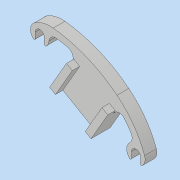
# Autodesk Inventor part: USBBreakoutHolder
Saved by Autodesk Inventor 2017 (Build 210142000, 142)
## iProperties
Created: 2019-07-16
Part Number: USBBreakoutHolder
Material: Generic
Document SubType Name: Modeling
Designer: techn
Density: 1 g/cm^3
Appearance: Default
Author: techn
Autodesk Inventor part; units mm, degrees
ref_plane "YZ Plane" through (0, 0, 0) normal (1, 0, 0) x (0, 1, 0)
ref_plane "XZ Plane" through (0, 0, 0) normal (0, 1, 0) x (-1, 0, 0)
ref_plane "XY Plane" through (0, 0, 0) normal (0, 0, 1) x (1, 0, 0)
sketch "Sketch1" plane through (0, 0, 0) normal (0, 0, 1) x (1, 0, 0)
  arc A0 (1.7145, 0) -> (-1.7145, 0) centre (0, 0) ccw
  arc A1 (38.0096, -20.955) -> (34.5806, -20.955) centre (36.2951, -20.955) ccw
  line L0 (0, 0) -> (36.5724, 0) construction
  line L1 (-1.7145, 0) -> (-1.7145, -3.0427)
  line L2 (1.7145, 0) -> (1.7145, -3.0427)
  line L3 (34.5806, -20.955) -> (34.5806, -23.9977)
  line L4 (38.0096, -20.955) -> (38.0096, -23.9977)
  line L5 (0, 0) -> (0, -41.91) construction
  arc A2 (29.1702, -5.2325) -> (5.0807, 4.6768) centre (0, -41.91) ccw
  arc A3 (5.0807, 4.6768) -> (-2.0016, 2.862) centre (3.9541, -5.6536) ccw
  arc A4 (39.5833, -19.7781) -> (29.1702, -5.2325) centre (8.8547, -30.7765) ccw
  arc A5 (4.8053, 2.1517) -> (2.7829, 2.1102) centre (3.9541, -5.6536) ccw
  arc A6 (27.5892, -7.2205) -> (4.8053, 2.1517) centre (0, -41.91) ccw
  arc A7 (35.8607, -17.4896) -> (27.5892, -7.2205) centre (8.8547, -30.7765) ccw
  arc A8 (35.8607, -17.4896) -> (34.5806, -23.9977) centre (36.2951, -20.955) ccw
  arc A9 (38.0096, -23.9977) -> (39.5833, -19.7781) centre (36.2951, -20.955) ccw
  arc A10 (-2.0016, 2.862) -> (-1.7145, -3.0427) centre (0, 0) ccw
  arc A11 (1.7145, -3.0427) -> (2.7829, 2.1102) centre (0, 0) ccw
  line L6 (0, 0) -> (36.2951, -20.955) construction
  line L7 (12.8786, -1.5696) -> (6.5286, -12.5681)
  line L8 (6.5286, -12.5681) -> (22.1465, -21.5851)
  line L9 (22.1465, -21.5851) -> (28.4965, -10.5866)
  line L10 (28.4965, -10.5866) -> (12.8786, -1.5696)
  line L11 (28.4965, -10.5866) -> (36.2951, -20.955) construction
  line L12 (12.8786, -1.5696) -> (0, 0) construction
  line L13 (12.8786, -1.5696) -> (13.8891, 0.1806)
  line L14 (28.4965, -10.5866) -> (29.4898, -8.8662)
  line L15 (15.0783, -2.8396) -> (8.7283, -13.8381)
  line L16 (26.2968, -9.3166) -> (19.9468, -20.3151)
  dimension "d0" = 3.429
  dimension "d1" = 30
  dimension "d3" = 41.91
  dimension "d4" = 93.726
  dimension "d6" = 2.54
  dimension "d7" = 5.08
  dimension "d8" = 18.034
  dimension "d9" = 41.91
  dimension "d10" = 6.985
  dimension "d11" = 12.7
  dimension "d12" = 2.54
  dimension "d13" = 2.54
  dimension "d14" = 3.429
  dimension "d15" = 3.4925
  constraints: 34 end point, 26 point on circle, 12 centre point, 8 tangent, 6 parallel, 5 point on line, 4 coincident, 2 collinear, 2 equal length, 2 equal radius, 2 perpendicular, 2 vertical, 1 horizontal
  measures "d0" diameter of A0
  measures "d3" distance of L5.start L5.end
  measures "d4" diameter of A2
  measures "d6" radial gap between concentric circles of A2 A6
  measures "d7" distance between parallel lines of L10 L6
  measures "d8" distance between parallel lines of L7 L9
  measures "d9" distance of L5.start L6.end
  measures "d10" diameter of A9
  measures "d11" distance of L8.end L9.end
  measures "d12" distance between parallel lines of L7 L15
  measures "d13" distance between parallel lines of L16 L9
  measures "d14" distance between parallel lines of L3 L4
  measures "d15" radius of A10
extrude "Extrusion1" add sketch "Sketch1" along normal blind 4.445
fillet "Fillet1" radius 2.54 4 edges at (2.7829, 2.1102, 2.2225) (35.8607, -17.4896, 2.2225) (29.4898, -8.8662, 2.2225) (13.8891, 0.1806, 2.2225)
fillet "Fillet2" radius 0.381 4 edges at (-1.7145, -3.0427, 2.2225) (1.7145, -3.0427, 2.2225) (34.5806, -23.9977, 2.2225) (38.0096, -23.9977, 2.2225)
extrude "Extrusion2" add sketch "Sketch1" along normal blind 7.239 contours L10 L15 L8 L7 | L9 L8 L16 L10
body "Solid1"
